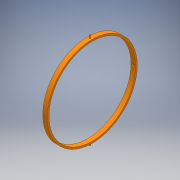
# Autodesk Inventor part: Middle Ring
Saved by Autodesk Inventor 2018 (Build 220112000, 112)
## iProperties
Created: 2018-03-07
Part Number: Middle Ring
Material: Generic
Document SubType Name: Modeling
Designer: sterl
Density: 1 g/cm^3
Appearance: Orange
Author: sterl
Autodesk Inventor part; units mm, degrees
ref_plane "YZ Plane" through (0, 0, 0) normal (1, 0, 0) x (0, 1, 0)
sketch "Sketch1" plane through (0, 0, 0) normal (1, 0, 0) x (0, 1, 0)
  circle A0 centre (0, 0) radius 100
  circle A1 centre (0, 0) radius 96
  dimension "d0" = 200
  dimension "d1" = 192
  constraints: 2 centre point, 2 coincident
  measures "d0" diameter of A0
  measures "d1" diameter of A1
extrude "Extrusion1" add sketch "Sketch1" along normal blind 10
ref_plane "Work Plane1" through (0, 100, 0) normal (0, 1, 0) x (-1, 0, 0)
sketch "Sketch2" plane through (0, 100, 0) normal (0, 1, 0) x (-1, 0, 0)
  line L0 (-10, 100) -> (-10, -100) projected
  line L1 (0, -100) -> (0, 100) projected
  line L2 (0, 0) -> (-10, 0)
  line L3 (-10, 100) -> (-10, -100) projected
  circle A0 centre (-5, 0) radius 2
  dimension "d4" = 4
  constraints: 2 end point, 2 midpoint, 1 centre point
  measures "d4" diameter of A0
extrude "Extrusion2" cut sketch "Sketch2" against normal blind 206.5
ref_plane "Work Plane2" through (0, 96, 0) normal (0, 1, 0) x (-1, 0, 0)
sketch "Sketch3" plane through (0, 96, 0) normal (0, 1, 0) x (-1, 0, 0)
  spline S0 degree 7 poles (-3, 0) (-3, 0.2763) (-3.0445, 0.5448) (-3.1291, 0.7973) (-3.2476, 1.027) (-3.3925, 1.2289) (-3.555, 1.4003) (-3.8877, 1.6755) (-4.0613, 1.7855) (-4.2426, 1.8721) (-4.4288, 1.9362) (-4.6182, 1.9787) (-4.809, 2) (-5.191, 2) (-5.3819, 1.9787) (-5.5712, 1.9362) (-5.7574, 1.8721) (-5.9387, 1.7855) (-6.1123, 1.6755) (-6.401, 1.4366) (-6.5214, 1.3168) (-6.6331, 1.1813) (-6.7335, 1.0306) (-6.8195, 0.8655) (-6.8884, 0.6871) (-6.9983, 0.2593) (-7.0264, 0.008) (-7.0168, -0.2475) (-6.9691, -0.4971) (-6.8869, -0.7312) (-6.7781, -0.9418) (-6.544, -1.2863) (-6.4193, -1.4299) (-6.2837, -1.555) (-6.1398, -1.6621) (-5.9897, -1.752) (-5.8351, -1.825) (-5.4467, -1.9649) (-5.2091, -2.0131) (-4.9685, -2.0281) (-4.7277, -2.0103) (-4.4896, -1.9594) (-4.2575, -1.8741) (-3.8074, -1.6267) (-3.5817, -1.4571) (-3.3742, -1.2407) (-3.1993, -0.9792) (-3.0704, -0.6784) (-3, -0.3473) (-3, 0) knots 0 0 0 0 0 0 0 0 0.126944 0.126944 0.126944 0.126944 0.126944 0.126944 0.248208 0.248208 0.248208 0.248208 0.248208 0.248208 0.369476 0.369476 0.369476 0.369476 0.369476 0.369476 0.463636 0.463636 0.463636 0.463636 0.463636 0.463636 0.581789 0.581789 0.581789 0.581789 0.581789 0.581789 0.686832 0.686832 0.686832 0.686832 0.686832 0.686832 0.840597 0.840597 0.840597 0.840597 0.840597 0.840597 1 1 1 1 1 1 1 1 projected
  line L0 (-7, 0) -> (-3, 0)
  circle A0 centre (-5, 0) radius 3
  point P0 (0, 0)
  dimension "d7" = 6
  constraints: 2 end point, 1 centre point, 1 horizontal, 1 midpoint, 3 other
  measures "d7" diameter of A0
extrude "Extrusion3" cut sketch "Sketch3" along normal mid plane 5
mirror "Mirror1" about plane through (0, 0, 0) normal (0, 1, 0) of "Extrusion3"
ref_plane "Work Plane3" through (0, 0, -100) normal (0, 0, 1) x (1, 0, 0)
sketch "Sketch4" plane through (0, 0, -100) normal (0, 0, 1) x (1, 0, 0)
  line L0 (10, -100) -> (10, 100) projected
  line L1 (0, 100) -> (0, -100) projected
  line L2 (0, 0) -> (10, 0)
  circle A0 centre (5, 0) radius 1.5
  dimension "d10" = 3
  constraints: 2 end point, 2 midpoint, 1 centre point
  measures "d10" diameter of A0
extrude "Extrusion4" add sketch "Sketch4" along normal mid plane 12
mirror "Mirror2" about plane through (0, 0, 0) normal (0, 0, 1) of "Extrusion4"
sketch "Sketch5" plane through (0, 0, 0) normal (-1, 0, 0) x (0, 0, 1)
  circle A0 centre (0, 0) radius 96 projected
extrude "Extrusion5" cut sketch "Sketch5" against normal blind 12
body "Solid1"
